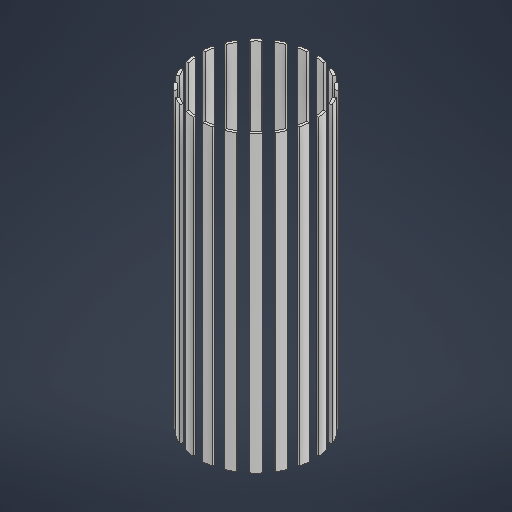
# Autodesk Inventor part: bandsbottomroller
Saved by Autodesk Inventor 2026.1 (Build 301233000, 233)
## iProperties
Created: 2025-08-08
Part Number: bandsbottomroller
Material: Generic
Document SubType Name: Modeling
Designer: roejo
Density: 1 g/cm^3
Appearance: Default
Author: roejo
Autodesk Inventor part; units mm, degrees
ref_plane "YZ Plane" through (0, 0, 0) normal (1, 0, 0) x (0, 1, 0)
ref_plane "XZ Plane" through (0, 0, 0) normal (0, 1, 0) x (-1, 0, 0)
ref_plane "XY Plane" through (0, 0, 0) normal (0, 0, 1) x (1, 0, 0)
sketch "Sketch1" plane through (0, 0, 0) normal (0, 1, 0) x (-1, 0, 0)
  circle A0 centre (0, 0) radius 36.5125
  dimension "d0" = 73.025
  constraints: 1 centre point, 1 coincident
  measures "d0" diameter of A0
extrude "Extrusion1" add sketch "Sketch1" along normal blind 184.15
sketch "Sketch2" plane through (0, 184.15, 0) normal (0, 1, 0) x (1, 0, 0)
  circle A0 centre (0, 0) radius 34.925
  dimension "d3" = 69.85
  constraints: 1 centre point, 1 coincident
  measures "d3" diameter of A0
extrude "Extrusion2" cut sketch "Sketch2" against normal through all
sketch "Sketch3" plane through (0, 184.15, 0) normal (0, 1, 0) x (1, 0, 0)
  line L0 (-31.75, -2.8575) -> (-37.465, -2.8575)
  line L1 (-37.465, -2.8575) -> (-37.465, 2.8575)
  line L2 (-37.465, 2.8575) -> (-31.75, 2.8575)
  line L3 (-31.75, 2.8575) -> (-31.75, -2.8575)
  circle A0 centre (0, 0) radius 36.5125 projected
  line L4 (-29.313, -12.5289) -> (-34.7483, -14.295)
  line L5 (-34.7483, -14.295) -> (-36.5143, -8.8597)
  line L6 (-36.5143, -8.8597) -> (-31.0791, -7.0936)
  line L7 (-31.0791, -7.0936) -> (-29.313, -12.5289)
  line L8 (-24.0067, -20.9739) -> (-28.6302, -24.3331)
  line L9 (-28.6302, -24.3331) -> (-31.9894, -19.7096)
  line L10 (-31.9894, -19.7096) -> (-27.3659, -16.3504)
  line L11 (-27.3659, -16.3504) -> (-24.0067, -20.9739)
  line L12 (-16.3504, -27.3659) -> (-19.7096, -31.9894)
  line L13 (-19.7096, -31.9894) -> (-24.3331, -28.6302)
  line L14 (-24.3331, -28.6302) -> (-20.9739, -24.0067)
  line L15 (-20.9739, -24.0067) -> (-16.3504, -27.3659)
  line L16 (-7.0936, -31.0791) -> (-8.8597, -36.5143)
  line L17 (-8.8597, -36.5143) -> (-14.295, -34.7483)
  line L18 (-14.295, -34.7483) -> (-12.5289, -29.313)
  line L19 (-12.5289, -29.313) -> (-7.0936, -31.0791)
  line L20 (2.8575, -31.75) -> (2.8575, -37.465)
  line L21 (2.8575, -37.465) -> (-2.8575, -37.465)
  line L22 (-2.8575, -37.465) -> (-2.8575, -31.75)
  line L23 (-2.8575, -31.75) -> (2.8575, -31.75)
  line L24 (12.5289, -29.313) -> (14.295, -34.7483)
  line L25 (14.295, -34.7483) -> (8.8597, -36.5143)
  line L26 (8.8597, -36.5143) -> (7.0936, -31.0791)
  line L27 (7.0936, -31.0791) -> (12.5289, -29.313)
  line L28 (20.9739, -24.0067) -> (24.3331, -28.6302)
  line L29 (24.3331, -28.6302) -> (19.7096, -31.9894)
  line L30 (19.7096, -31.9894) -> (16.3504, -27.3659)
  line L31 (16.3504, -27.3659) -> (20.9739, -24.0067)
  line L32 (27.3659, -16.3504) -> (31.9894, -19.7096)
  line L33 (31.9894, -19.7096) -> (28.6302, -24.3331)
  line L34 (28.6302, -24.3331) -> (24.0067, -20.9739)
  line L35 (24.0067, -20.9739) -> (27.3659, -16.3504)
  line L36 (31.0791, -7.0936) -> (36.5143, -8.8597)
  line L37 (36.5143, -8.8597) -> (34.7483, -14.295)
  line L38 (34.7483, -14.295) -> (29.313, -12.5289)
  line L39 (29.313, -12.5289) -> (31.0791, -7.0936)
  line L40 (31.75, 2.8575) -> (37.465, 2.8575)
  line L41 (37.465, 2.8575) -> (37.465, -2.8575)
  line L42 (37.465, -2.8575) -> (31.75, -2.8575)
  line L43 (31.75, -2.8575) -> (31.75, 2.8575)
  line L44 (29.313, 12.5289) -> (34.7483, 14.295)
  line L45 (34.7483, 14.295) -> (36.5143, 8.8597)
  line L46 (36.5143, 8.8597) -> (31.0791, 7.0936)
  line L47 (31.0791, 7.0936) -> (29.313, 12.5289)
  line L48 (24.0067, 20.9739) -> (28.6302, 24.3331)
  line L49 (28.6302, 24.3331) -> (31.9894, 19.7096)
  line L50 (31.9894, 19.7096) -> (27.3659, 16.3504)
  line L51 (27.3659, 16.3504) -> (24.0067, 20.9739)
  line L52 (16.3504, 27.3659) -> (19.7096, 31.9894)
  line L53 (19.7096, 31.9894) -> (24.3331, 28.6302)
  line L54 (24.3331, 28.6302) -> (20.9739, 24.0067)
  line L55 (20.9739, 24.0067) -> (16.3504, 27.3659)
  line L56 (7.0936, 31.0791) -> (8.8597, 36.5143)
  line L57 (8.8597, 36.5143) -> (14.295, 34.7483)
  line L58 (14.295, 34.7483) -> (12.5289, 29.313)
  line L59 (12.5289, 29.313) -> (7.0936, 31.0791)
  line L60 (-2.8575, 31.75) -> (-2.8575, 37.465)
  line L61 (-2.8575, 37.465) -> (2.8575, 37.465)
  line L62 (2.8575, 37.465) -> (2.8575, 31.75)
  line L63 (2.8575, 31.75) -> (-2.8575, 31.75)
  line L64 (-12.5289, 29.313) -> (-14.295, 34.7483)
  line L65 (-14.295, 34.7483) -> (-8.8597, 36.5143)
  line L66 (-8.8597, 36.5143) -> (-7.0936, 31.0791)
  line L67 (-7.0936, 31.0791) -> (-12.5289, 29.313)
  line L68 (-20.9739, 24.0067) -> (-24.3331, 28.6302)
  line L69 (-24.3331, 28.6302) -> (-19.7096, 31.9894)
  line L70 (-19.7096, 31.9894) -> (-16.3504, 27.3659)
  line L71 (-16.3504, 27.3659) -> (-20.9739, 24.0067)
  line L72 (-27.3659, 16.3504) -> (-31.9894, 19.7096)
  line L73 (-31.9894, 19.7096) -> (-28.6302, 24.3331)
  line L74 (-28.6302, 24.3331) -> (-24.0067, 20.9739)
  line L75 (-24.0067, 20.9739) -> (-27.3659, 16.3504)
  line L76 (-31.0791, 7.0936) -> (-36.5143, 8.8597)
  line L77 (-36.5143, 8.8597) -> (-34.7483, 14.295)
  line L78 (-34.7483, 14.295) -> (-29.313, 12.5289)
  line L79 (-29.313, 12.5289) -> (-31.0791, 7.0936)
  circle A1 centre (0, 0) radius 34.925 projected
  point P0 (-36.5125, 0)
  point P1 (-34.7255, -11.283)
  point P2 (-29.5392, -21.4615)
  point P3 (-21.4615, -29.5392)
  point P4 (-11.283, -34.7255)
  point P5 (0, -36.5125)
  point P6 (11.283, -34.7255)
  point P7 (21.4615, -29.5392)
  point P8 (29.5392, -21.4615)
  point P9 (34.7255, -11.283)
  point P10 (36.5125, 0)
  point P11 (34.7255, 11.283)
  point P12 (29.5392, 21.4615)
  point P13 (21.4615, 29.5392)
  point P14 (11.283, 34.7255)
  point P15 (0, 36.5125)
  point P16 (-11.283, 34.7255)
  point P17 (-21.4615, 29.5392)
  point P18 (-29.5392, 21.4615)
  point P19 (-34.7255, 11.283)
  dimension "d6" = 5.715
  dimension "d7" = 5.715
  dimension "d8" = 2.8575
  dimension "d13" = 360
  dimension "d15" = 2.54
  constraints: 160 end point, 2 parallel, 1 horizontal, 1 horizontal alignment, 1 perpendicular, 182 other
  measures "d6" distance of L1.end L2.end
  measures "d7" distance of L0.end L1.end
  measures "d8" distance from line of L2 point (-36.513, 0)
  measures "d15" distance edge to line of A1 L1
extrude "Extrusion3" cut sketch "Sketch3" against normal through all contours L0 A1 L2 L3 | L0 A0 L2 A1 | L0 L1 L2 A0 | A1 L4 A0 L6 | L6 L7 L4 A1 | A0 L4 L5 L6 | A1 L78 L79 L76 | L76 A0 L78 A1 | L76 L77 L78 A0 | A1 L8 A0 L10 | L10 L11 L8 A1 | A0 L8 L9 L10 | A1 L74 L75 L72 | L72 A0 L74 A1 | L72 L73 L74 A0 | A1 L12 A0 L14 | L14 L15 L12 A1 | A0 L12 L13 L14 | A1 L70 L71 L68 | L68 A0 L70 A1 | L68 L69 L70 A0 | A1 L16 A0 L18 | L18 L19 L16 A1 | A0 L16 L17 L18 | A1 L66 L67 L64 | L64 A0 L66 A1 | L64 L65 L66 A0 | A1 L20 A0 L22 | L22 L23 L20 A1 | A0 L20 L21 L22 | A1 L62 L63 L60 | L60 A0 L62 A1 | L60 L61 L62 A0 | A1 L24 A0 L26 | L26 L27 L24 A1 | A0 L24 L25 L26 | A1 L58 L59 L56 | L56 A0 L58 A1 | L56 L57 L58 A0 | A1 L28 A0 L30 | L30 L31 L28 A1 | A0 L28 L29 L30 | A1 L54 L55 L52 | L52 A0 L54 A1 | L52 L53 L54 A0 | A1 L32 A0 L34 | L34 L35 L32 A1 | A0 L32 L33 L34 | A1 L50 L51 L48 | L48 A0 L50 A1 | L48 L49 L50 A0 | A1 L36 A0 L38 | L38 L39 L36 A1 | A0 L36 L37 L38 | A1 L46 L47 L44 | L44 A0 L46 A1 | L44 L45 L46 A0 | A1 L40 A0 L42 | L42 L43 L40 A1 | A0 L40 L41 L42
body "Solid1"
